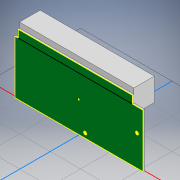
# Autodesk Inventor part: TL-SF1005D_pcb
Saved by Autodesk Inventor 2022 (Build 260153000, 153)
## iProperties
Created: 2023-02-17
Part Number: TL-SF1005D_pcb
Material: Типовые
Document SubType Name: Modeling
Designer: Иван Петров
Density: 1 g/cm^3
Appearance: По умолчанию
Author: Иван Петров
Autodesk Inventor part; units mm, degrees
ref_plane "YZ Plane" through (0, 0, 0) normal (1, 0, 0) x (0, 1, 0)
ref_plane "XZ Plane" through (0, 0, 0) normal (0, 1, 0) x (-1, 0, 0)
ref_plane "XY Plane" through (0, 0, 0) normal (0, 0, 1) x (1, 0, 0)
sketch "Эскиз1" plane through (0, 0, 0) normal (0, 0, 1) x (1, 0, 0)
  line L0 (-42, -20) -> (42, -20)
  line L1 (42, -20) -> (42, 20)
  line L2 (42, 20) -> (-42, 20)
  line L3 (-42, 20) -> (-42, -20)
  line L4 (-42, -20) -> (42, 20) construction
  line L5 (42, -20) -> (-42, 20) construction
  line L6 (-42, 20) -> (-40, 20)
  line L7 (-40, 20) -> (-40, 15)
  line L8 (-40, 15) -> (-42, 15)
  line L9 (-42, 15) -> (-42, 20)
  line L10 (42, 20) -> (35, 20)
  line L11 (35, 20) -> (35, 15)
  line L12 (35, 15) -> (42, 15)
  line L13 (42, 15) -> (42, 20)
  point P0 (0, 0)
  dimension "d0" = 84
  dimension "d1" = 40
  dimension "d3" = 5
  dimension "d4" = 2
  dimension "d20" = 75
  constraints: 28 end point, 6 parallel, 3 horizontal, 3 perpendicular, 2 midpoint, 1 horizontal alignment, 1 point on line
  measures "d0" distance of L2.end L1.end
  measures "d1" distance of L1.end L0.end
  measures "d3" distance between parallel lines of L12 L2
  measures "d4" distance between parallel lines of L3 L7
  measures "d20" distance between parallel lines of L7 L11
extrude "Выдавливание1" add sketch "Эскиз1" along normal blind 1 contours L3 L8 L7 L2 L11 L12 L1 L0
sketch "Эскиз2" plane through (0, 0, 0) normal (0, 0, -1) x (-1, 0, 0)
  line L0 (40, 8.5) -> (-35, 8.5)
  line L1 (-35, 8.5) -> (-35, 23.5)
  line L2 (-35, 23.5) -> (40, 23.5)
  line L3 (40, 23.5) -> (40, 8.5)
  line L4 (-35, 20) -> (40, 20) projected
  point P0 (0, 0)
  point P1 (40, 15)
  point P2 (-35, 15)
  dimension "d7" = 3.5
  dimension "d8" = 15
  constraints: 8 end point, 2 parallel, 2 point on line, 1 horizontal, 1 perpendicular
  measures "d7" distance between parallel lines of L2 L4
  measures "d8" distance between parallel lines of L2 L0
extrude "Выдавливание2" add sketch "Эскиз2" along normal blind 13.5
sketch "Эскиз3" plane through (0, 0, 1) normal (0, 0, 1) x (1, 0, 0)
  circle A0 centre (4, -17) radius 1
  line L0 (-42, -20) -> (42, -20) projected
  line L1 (-42, 15) -> (-42, -20) projected
  circle A1 centre (38, 0) radius 1
  line L2 (42, 15) -> (35, 15) projected
  line L3 (42, -20) -> (42, 15) projected
  point P0 (0, 0)
  dimension "d11" = 2
  dimension "d12" = 3
  dimension "d13" = 46
  dimension "d14" = 2
  dimension "d15" = 15
  dimension "d16" = 4
  constraints: 2 centre point
  measures "d11" diameter of A0
  measures "d12" distance from line of L0 A0.centre
  measures "d13" distance from line of L1 A0.centre
  measures "d14" diameter of A1
  measures "d15" distance from line of L2 A1.centre
  measures "d16" distance from line of L3 A1.centre
extrude "Выдавливание3" cut sketch "Эскиз3" against normal through all
sketch "Эскиз4" plane through (0, 0, 1) normal (0, 0, 1) x (1, 0, 0)
  circle A0 centre (38, 0) radius 1 projected
  circle A1 centre (4, -17) radius 1 projected
  line L0 (42, -20) -> (42, 15) projected
  line L1 (42, 15) -> (35, 15) projected
  line L2 (35, 15) -> (35, 20) projected
  line L3 (35, 20) -> (-40, 20) projected
  line L4 (-40, 20) -> (-40, 15) projected
  line L5 (-40, 15) -> (-42, 15) projected
  line L6 (-42, 15) -> (-42, -20) projected
  line L7 (-42, -20) -> (42, -20) projected
  line L8 (42, 15) -> (35, 15) projected
  line L9 (-40, 15) -> (35, 15)
  point P0 (0, 0)
  constraints: 2 end point, 1 horizontal
